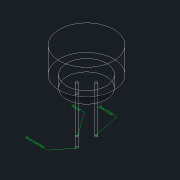
# Autodesk Inventor part: МП41А
Saved by Autodesk Inventor 2021.2 (Build 252289000, 289)
## iProperties
Created: 2022-04-11
Part Number: МП41А
Material: Типовые
Document SubType Name: Modeling
Designer: Александр
Density: 1 g/cm^3
Appearance: По умолчанию
Author: Александр
Autodesk Inventor part; units mm, degrees
ref_plane "YZ Plane" through (0, 0, 0) normal (1, 0, 0) x (0, 1, 0)
ref_plane "XZ Plane" through (0, 0, 0) normal (0, 1, 0) x (-1, 0, 0)
ref_plane "XY Plane" through (0, 0, 0) normal (0, 0, 1) x (1, 0, 0)
sketch "Эскиз1" plane through (0, 0, 0) normal (0, 1, 0) x (-1, 0, 0)
  circle A0 centre (0, 0) radius 5.85
  dimension "d2" = 11.7
  constraints: 1 centre point, 1 coincident
  measures "d2" diameter of A0
extrude "Выдавливание1" add sketch "Эскиз1" along normal blind 5.5
sketch "Эскиз2" plane through (0, 0, 0) normal (0, -1, 0) x (1, 0, 0)
  circle A0 centre (0, 0) radius 4.25
  dimension "d5" = 8.5
  constraints: 1 centre point, 1 coincident
  measures "d5" diameter of A0
extrude "Выдавливание2" add sketch "Эскиз2" along normal blind 2.5
sketch "Эскиз3" plane through (0, -2.5, 0) normal (0, -1, 0) x (1, 0, 0)
  circle A0 centre (0, 0) radius 2.1 construction
  circle A1 centre (0, 2.1) radius 0.25
  circle A2 centre (-2.1, 0) radius 0.25
  circle A3 centre (0, -2.1) radius 0.25
  dimension "d6" = 4.2
  dimension "d7" = 0.5
  dimension "d8" = 0.5
  dimension "d9" = 0.5
  constraints: 4 centre point, 3 point on circle, 1 coincident
  measures "d6" diameter of A0
  measures "d7" diameter of A1
  measures "d8" diameter of A2
  measures "d9" diameter of A3
extrude "Выдавливание3" add sketch "Эскиз3" along normal blind 10 separate body contours A1
extrude "Выдавливание4" add sketch "Эскиз3" along normal blind 10 separate body contours A2
extrude "Выдавливание5" add sketch "Эскиз3" along normal blind 10 separate body contours A3
